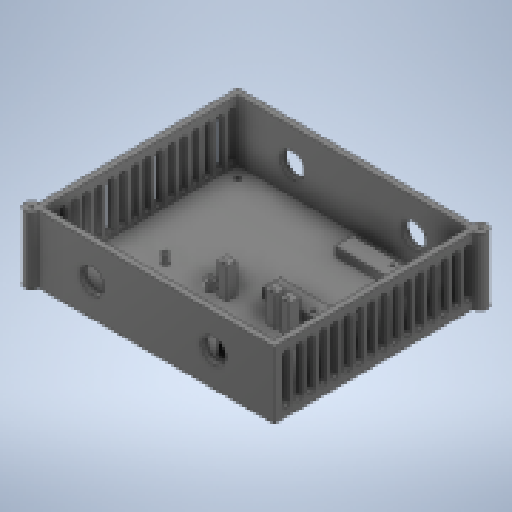
# Autodesk Inventor part: Power Box (12V)
Saved by Autodesk Inventor 2026.2 (Build 302298010, 298A)
## iProperties
Created: 2026-05-01
Part Number: Power Box (12V)
Material: ABS Plastic
Document SubType Name: Modeling
Designer: chanh
Density: 1.06 g/cm^3
Appearance: Smooth - White
Author: chanh
Autodesk Inventor part; units mm, degrees
ref_plane "YZ Plane" through (0, 0, 0) normal (1, 0, 0) x (0, 1, 0)
ref_plane "XZ Plane" through (0, 0, 0) normal (0, 1, 0) x (-1, 0, 0)
ref_plane "XY Plane" through (0, 0, 0) normal (0, 0, 1) x (1, 0, 0)
sketch "Sketch1" plane through (0, 0, 0) normal (0, 1, 0) x (-1, 0, 0)
  line L0 (100, 85) -> (-100, 85)
  line L1 (-100, 85) -> (-100, -85)
  line L2 (-100, -85) -> (100, -85)
  line L3 (100, -85) -> (100, 85)
  line L4 (100, 85) -> (-100, -85) construction
  line L5 (-100, 85) -> (100, -85) construction
  point P0 (0, 0)
  dimension "d0" = 200
  dimension "d1" = 170
  constraints: 12 end point, 2 midpoint, 2 parallel, 1 horizontal, 1 perpendicular
  measures "d0" distance of L2.end L1.end
  measures "d1" distance of L0.end L1.end
extrude "Extrusion1" add sketch "Sketch1" along normal blind 55
shell "Shell1" thickness 5 removed faces 1 at (33.3333, 55, 28.3333)
sketch "Sketch2" plane through (-95, 5, -80) normal (0, 1, 0) x (1, 0, 0)
  line L0 (141, -100) -> (181, -100) construction
  line L1 (181, -100) -> (181, -140) construction
  line L2 (181, -140) -> (141, -140) construction
  line L3 (141, -140) -> (141, -100) construction
  line L4 (141, -100) -> (181, -140) construction
  line L5 (181, -100) -> (141, -140) construction
  line L6 (89, -100) -> (129, -100) construction
  line L7 (129, -100) -> (129, -140) construction
  line L8 (129, -140) -> (89, -140) construction
  line L9 (89, -140) -> (89, -100) construction
  line L10 (89, -100) -> (129, -140) construction
  line L11 (129, -100) -> (89, -140) construction
  line L12 (190, -160) -> (190, 0) projected
  line L13 (190, 0) -> (0, 0) projected
  line L14 (0, 0) -> (0, -160) projected
  line L15 (0, -160) -> (190, -160) projected
  line L16 (40, -100) -> (77, -100) construction
  line L17 (77, -100) -> (77, -137) construction
  line L18 (77, -137) -> (40, -137) construction
  line L19 (40, -137) -> (40, -100) construction
  line L20 (40, -100) -> (77, -137) construction
  line L21 (77, -100) -> (40, -137) construction
  point P0 (95, -80)
  point P1 (161, -120)
  point P2 (109, -120)
  point P3 (58.5, -118.5)
  dimension "d5" = 40
  dimension "d6" = 40
  dimension "d7" = 12
  dimension "d8" = 20
  dimension "d9" = 9
  dimension "d10" = 37
  dimension "d11" = 37
  dimension "d12" = 12
  constraints: 36 end point, 6 midpoint, 6 parallel, 5 perpendicular, 3 horizontal, 1 collinear, 1 horizontal alignment
  measures "d5" distance of L3.end L1.start
  measures "d6" distance of L10.start L7.start
  measures "d7" distance between parallel lines of L3 L7
  measures "d8" distance between parallel lines of L2 L15
  measures "d9" distance between parallel lines of L12 L1
  measures "d10" distance of L17.end L18.end
  measures "d11" distance of L16.end L17.end
  measures "d12" distance between parallel lines of L9 L17
sketch "Sketch3" plane through (-95, 5, -80) normal (0, 1, 0) x (1, 0, 0)
  circle A0 centre (89, -140) radius 4
  circle A1 centre (129, -140) radius 4
  circle A2 centre (141, -140) radius 4
  circle A3 centre (181, -140) radius 4
  line L0 (85, -94) -> (93, -94)
  line L1 (93, -94) -> (93, -102)
  line L2 (93, -102) -> (85, -102)
  line L3 (85, -102) -> (85, -94)
  line L4 (85, -94) -> (93, -102) construction
  line L5 (93, -94) -> (85, -102) construction
  line L6 (125, -94) -> (133, -94)
  line L7 (133, -94) -> (133, -102)
  line L8 (133, -102) -> (125, -102)
  line L9 (125, -102) -> (125, -94)
  line L10 (125, -94) -> (133, -102) construction
  line L11 (133, -94) -> (125, -102) construction
  line L12 (137, -94) -> (145, -94)
  line L13 (145, -94) -> (145, -102)
  line L14 (145, -102) -> (137, -102)
  line L15 (137, -102) -> (137, -94)
  line L16 (137, -94) -> (145, -102) construction
  line L17 (145, -94) -> (137, -102) construction
  line L18 (177, -94) -> (185, -94)
  line L19 (185, -94) -> (185, -102)
  line L20 (185, -102) -> (177, -102)
  line L21 (177, -102) -> (177, -94)
  line L22 (177, -94) -> (185, -102) construction
  line L23 (185, -94) -> (177, -102) construction
  line L24 (133, -94) -> (137, -94)
  line L25 (137, -102) -> (133, -102)
  line L26 (129, -136) -> (141, -136)
  line L27 (129, -144) -> (141, -144)
  point P0 (95, -80)
  point P1 (181, -100)
  point P2 (141, -100)
  point P3 (129, -100)
  point P4 (89, -100)
  point P5 (89, -98)
  point P6 (129, -98)
  point P7 (141, -98)
  point P8 (181, -98)
  dimension "d13" = 8
  dimension "d14" = 8
  dimension "d15" = 8
  dimension "d16" = 8
  dimension "d17" = 8
  dimension "d18" = 8
  dimension "d19" = 8
  dimension "d20" = 8
  dimension "d21" = 8
  dimension "d22" = 2
  dimension "d23" = 2
  dimension "d24" = 2
  dimension "d25" = 2
  constraints: 56 end point, 9 parallel, 8 midpoint, 4 centre point, 4 coincident, 4 horizontal, 4 perpendicular, 4 point on circle, 4 vertical alignment, 3 equal radius, 3 tangent
  measures "d13" diameter of A0
  measures "d14" distance of L1.end L2.end
  measures "d15" distance of L0.end L1.end
  measures "d16" distance of L7.end L8.end
  measures "d17" distance of L6.end L7.end
  measures "d18" distance of L14.start L14.end
  measures "d19" distance of L12.end L14.start
  measures "d20" distance of L20.start L20.end
  measures "d21" distance of L18.end L20.start
  measures "d22" distance from line of L2 point (89, -100)
  measures "d23" distance from line of point (129, -100) L8
  measures "d24" distance from line of point (141, -100) L14
  measures "d25" distance from line of point (181, -100) L20
extrude "Extrusion2" add sketch "Sketch3" along normal blind 25 contours A0 | A1 | A1 L26 A2 L27 | A2 | A3 | L0 L1 L2 L3 | L6 L7 L8 L9 | L12 L13 L14 L15 | L18 L19 L20 L21
sketch "Sketch4" plane through (-95, 30, -80) normal (0, 1, 0) x (1, 0, 0)
  point P0 (95, -80)
  point P1 (89, -100)
  point P2 (129, -100)
  point P3 (141, -100)
  point P4 (181, -100)
  point P5 (181, -140)
  point P6 (141, -140)
  point P7 (129, -140)
  point P8 (89, -140)
hole "Hole1" at (-6, 30, 20) at (34, 30, 20) at (46, 30, 20) at (86, 30, 20) at (86, 30, 60) at (46, 30, 60) at (34, 30, 60) at (-6, 30, 60) direction (0, -1, 0) diameter 2.7 depth 7
sketch "Sketch5" plane through (-95, 5, -80) normal (0, 1, 0) x (1, 0, 0)
  circle A0 centre (40, -137) radius 4
  circle A1 centre (77, -137) radius 4
  circle A2 centre (77, -100) radius 4
  circle A3 centre (40, -100) radius 3
  point P0 (95, -80)
  dimension "d35" = 8
  dimension "d36" = 8
  dimension "d37" = 8
  dimension "d38" = 6
  constraints: 4 centre point, 4 coincident
  measures "d35" diameter of A0
  measures "d36" diameter of A1
  measures "d37" diameter of A2
  measures "d38" diameter of A3
extrude "Extrusion3" add sketch "Sketch5" along normal blind 7
sketch "Sketch6" plane through (-18, 12, 20) normal (0, 1, 0) x (1, 0, 0)
  circle A0 centre (-37, 0) radius 3 projected
  circle A1 centre (-37, -37) radius 4 projected
  circle A2 centre (0, -37) radius 4 projected
  circle A3 centre (0, 0) radius 4 projected
  point P0 (18, 20)
hole "Hole2" at (-55, 12, 20) at (-18, 12, 20) at (-55, 12, 57) at (-18, 12, 57) direction (0, -1, 0) diameter 2.7 depth 7
sketch "Sketch7" plane through (-95, 5, -80) normal (0, 1, 0) x (1, 0, 0)
  line L0 (105, -10) -> (180, -10)
  line L1 (180, -10) -> (180, -85)
  line L2 (180, -85) -> (105, -85)
  line L3 (105, -85) -> (105, -10)
  line L4 (105, -10) -> (180, -85) construction
  line L5 (180, -10) -> (105, -85) construction
  line L6 (190, 0) -> (190, -160) projected
  line L7 (0, 0) -> (190, 0) projected
  line L8 (105, -25) -> (180, -25)
  line L9 (105, -70) -> (180, -70)
  point P0 (95, -80)
  point P1 (142.5, -47.5)
  point P2 (142.5, -25)
  dimension "d48" = 75
  dimension "d49" = 75
  dimension "d50" = 10
  dimension "d51" = 10
  dimension "d52" = 15
  dimension "d53" = 15
  constraints: 16 end point, 4 point on line, 3 midpoint, 3 perpendicular, 2 parallel, 1 horizontal
  measures "d48" distance of L1.end L2.end
  measures "d49" distance of L0.end L1.end
  measures "d50" distance between parallel lines of L6 L1
  measures "d51" distance between parallel lines of L7 L0
  measures "d52" distance from line of L0 point (142.5, -25)
  measures "d53" distance between parallel lines of L2 L9
extrude "Extrusion4" add sketch "Sketch7" along normal blind 7 contours L0 L1 L8 L3 | L9 L1 L2 L3
sketch "Sketch8" plane through (-95, 12, -80) normal (0, 1, 0) x (1, 0, 0)
  line L0 (105, -10) -> (105, -25) projected
  line L1 (105, -25) -> (180, -25) projected
  line L2 (180, -25) -> (180, -10) projected
  line L3 (180, -10) -> (105, -10) projected
  line L4 (180, -85) -> (180, -70) projected
  line L5 (180, -70) -> (105, -70) projected
  line L6 (105, -70) -> (105, -85) projected
  line L7 (105, -85) -> (180, -85) projected
  point P0 (95, -80)
  point P1 (142.5, -15)
  point P2 (142.5, -80)
  point P3 (142.5, -10)
  point P4 (180, -17.5)
  point P5 (180, -77.5)
  dimension "d56" = 5
  dimension "d57" = 5
  constraints: 3 midpoint, 2 vertical alignment
  measures "d56" distance from line of L3 point (142.5, -15)
  measures "d57" distance from line of L7 point (142.5, -80)
hole "Hole3" at (47.5, 12, -65) at (47.5, 12, 0) direction (0, -1, 0) diameter 3.7 depth 7
sketch "Sketch9" plane through (-100, 0, 85) normal (0, 0, 1) x (1, 0, 0)
  line L0 (0, 0) -> (200, 0) projected
  line L1 (200, 0) -> (200, 55) projected
  line L2 (0, 55) -> (200, 55) projected
  line L3 (0, 0) -> (0, 55) projected
  circle A0 centre (50, 27.5) radius 10
  circle A1 centre (150, 27.5) radius 10
  line L4 (50, 27.5) -> (150, 27.5) construction
  point P0 (100, 0)
  point P1 (100, 27.5)
  point P2 (100, 55)
  point P3 (0, 27.5)
  dimension "d65" = 20
  dimension "d66" = 20
  dimension "d67" = 100
  constraints: 3 midpoint, 2 centre point, 2 end point, 2 horizontal alignment, 1 perpendicular, 1 vertical alignment
  measures "d65" diameter of A1
  measures "d66" diameter of A0
  measures "d67" distance of L4.end L4.start
extrude "Extrusion5" cut sketch "Sketch9" against normal up to surface (5 mm away) contours A0 | A1
mirror "Mirror1" about plane through (0, 0, 0) normal (0, 0, 1) of "Extrusion5"
sketch "Sketch10" plane through (0, 55, 0) normal (0, 1, 0) x (1, 0, 0)
  line L0 (85, -5) -> (10, -5) projected
  line L1 (10, -5) -> (10, 10) projected
  line L2 (10, 10) -> (85, 10) projected
  line L3 (85, 10) -> (85, -5) projected
  line L4 (10, 70) -> (85, 70) projected
  line L5 (85, 70) -> (85, 55) projected
  line L6 (85, 55) -> (10, 55) projected
  line L7 (10, 55) -> (10, 70) projected
  circle A0 centre (-18, -57) radius 4 projected
  circle A1 centre (-55, -57) radius 4 projected
  circle A2 centre (-55, -20) radius 3 projected
  circle A3 centre (-18, -20) radius 4 projected
  line L8 (42, -22) -> (42, -14) projected
  line L9 (42, -14) -> (50, -14) projected
  line L10 (50, -14) -> (50, -22) projected
  line L11 (50, -22) -> (42, -22) projected
  circle A4 centre (86, -60) radius 4 projected
  line L12 (90, -14) -> (90, -22) projected
  line L13 (90, -22) -> (82, -22) projected
  line L14 (82, -22) -> (82, -14) projected
  line L15 (82, -14) -> (90, -14) projected
  line L16 (30, -22) -> (30, -14) projected
  line L17 (30, -14) -> (38, -14) projected
  line L18 (38, -14) -> (38, -22) projected
  line L19 (38, -22) -> (30, -22) projected
  arc A5 (34, -56) -> (34, -64) centre (34, -60) ccw projected
  line L20 (34, -56) -> (46, -56) projected
  arc A6 (46, -64) -> (46, -56) centre (46, -60) ccw projected
  line L21 (46, -64) -> (34, -64) projected
  circle A7 centre (-6, -60) radius 4 projected
  line L22 (-10, -22) -> (-10, -14) projected
  line L23 (-10, -14) -> (-2, -14) projected
  line L24 (-2, -14) -> (-2, -22) projected
  line L25 (-2, -22) -> (-10, -22) projected
  line L26 (95, -80) -> (95, 80) projected
  line L27 (95, 80) -> (-95, 80) projected
  line L28 (-95, 80) -> (-95, -80) projected
  line L29 (-95, -80) -> (95, -80) projected
  line L30 (0, 80) -> (0, -80) construction
  line L31 (-95, 0) -> (95, 0) construction
  point P0 (0, 0)
  point P1 (-85, 70)
  point P2 (-85, -70)
  point P3 (85, -70)
  dimension "d70" = 10
  dimension "d71" = 10
  constraints: 4 end point, 4 midpoint, 2 symmetric about line
  measures "d70" distance from line of L27 point (-85, 70)
  measures "d71" distance from line of L28 point (-85, 70)
hole "Hole4" at (-85, 55, -70) at (-85, 55, 70) at (85, 55, 70) direction (0, -1, 0) diameter 4.2 end through all
sketch "Sketch11" plane through (-95, 5, -80) normal (1, 0, 0) x (0, 0, -1)
  line L0 (-152, 40) -> (-152, 5)
  line L1 (-158, 5) -> (-158, 40)
  arc A0 (-152, 40) -> (-158, 40) centre (-155, 40) ccw
  arc A1 (-158, 5) -> (-152, 5) centre (-155, 5) ccw
  line L2 (-155, 40) -> (-155, 5) construction
  line L3 (-165, -5) -> (-165, 50) projected
  line L4 (5, 50) -> (-165, 50) projected
  point P0 (-80, -5)
  point P1 (-155, 22.5)
  point P2 (-165, 22.5)
  dimension "d79" = 35
  dimension "d80" = 6
  dimension "d81" = 10
  constraints: 6 end point, 4 point on circle, 4 tangent, 2 centre point, 2 midpoint, 1 horizontal alignment, 1 parallel, 1 vertical
  measures "d79" distance of L2.start L2.end
  measures "d80" distance between parallel lines of L0 L1
  measures "d81" distance from line of point (-155, 22.5) L3
extrude "Extrusion6" cut sketch "Sketch11" against normal through all
pattern_linear "Rectangular Pattern1" count 16 spacing 10 along (0, 0, -1) of "Extrusion6"
mirror "Mirror2" about plane through (0, 0, 0) normal (1, 0, 0) of "Extrusion6", "Rectangular Pattern1"
sketch "Sketch12" plane through (0, 55, 0) normal (0, 1, 0) x (1, 0, 0)
  line L0 (95, -80) -> (-95, -80) projected
  line L1 (-95, -80) -> (-95, 80) projected
  line L2 (-95, 80) -> (95, 80) projected
  line L3 (95, 80) -> (95, -80) projected
  line L4 (100, -85) -> (100, 85) projected
  line L5 (100, 85) -> (-100, 85) projected
  line L6 (-100, 85) -> (-100, -85) projected
  line L7 (-100, -85) -> (100, -85) projected
  circle A0 centre (100, 85) radius 6
  circle A1 centre (-100, -85) radius 6
  point P0 (0, 0)
  point P1 (94, 85)
  point P2 (100, 79)
  point P3 (-100, -79)
  point P4 (-94, -85)
  dimension "d87" = 12
  constraints: 2 centre point, 2 coincident, 1 equal radius
  measures "d87" diameter of A0
extrude "Extrusion7" add sketch "Sketch12" against normal up to surface (55 mm away) contours L4 L5 A0 | A1 L6 L7 picked at (102.6332, 87.9722) picked at (-103.8848, -84.1854)
sketch "Sketch13" plane through (0, 55, 0) normal (0, 1, 0) x (1, 0, 0)
  line L0 (95, -80) -> (-95, -80) projected
  line L1 (-95, -80) -> (-95, 80) projected
  line L2 (-95, 80) -> (95, 80) projected
  line L3 (95, 80) -> (95, -80) projected
  line L4 (100, -85) -> (100, 79) projected
  arc A0 (100, 79) -> (94, 85) centre (100, 85) ccw projected
  line L5 (94, 85) -> (-100, 85) projected
  line L6 (-100, 85) -> (-100, -79) projected
  arc A1 (-100, -79) -> (-94, -85) centre (-100, -85) ccw projected
  line L7 (-94, -85) -> (100, -85) projected
  point P0 (0, 0)
hole "Hole5" at (-100, 55, 85) at (100, 55, -85) direction (0, -1, 0) diameter 2.7 depth 8
equation "\"d68\" = d7"
body "Solid1"
